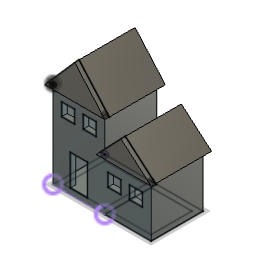
MMEZP_Domecek_3_Pokoje v1 (Autodesk Fusion 360 design; units mm, degrees)
Autodesk Fusion 360 part; units mm, degrees
sketch "Sketch1" plane through (0, 0, 0) normal (0, 1, 0) x (1, 0, 0)
  line L0 (0, 0) -> (30, 0)
  line L1 (30, 0) -> (30, -30)
  line L2 (30, -30) -> (0, -30)
  line L3 (0, -30) -> (0, 0)
  line L4 (3.2, -3.2) -> (26.8, -3.2)
  line L5 (26.8, -3.2) -> (26.8, -26.8)
  line L6 (26.8, -26.8) -> (3.2, -26.8)
  line L7 (3.2, -26.8) -> (3.2, -3.2)
  line L8 (30, 0) -> (56.8, 0)
  line L9 (56.8, 0) -> (56.8, -30)
  line L10 (56.8, -30) -> (30, -30)
  line L11 (30, -30) -> (30, 0)
  line L12 (30, -3.2) -> (53.6, -3.2)
  line L13 (53.6, -3.2) -> (53.6, -26.8)
  line L14 (53.6, -26.8) -> (30, -26.8)
  dimension "d7" = 30
  dimension "d8" = 30
  dimension "d9" = 3.2
  dimension "d10" = 3.2
  dimension "d11" = 3.2
  dimension "d12" = 3.2
  dimension "d13" = 26.8
  dimension "d14" = 30
  dimension "d15" = 3.2
  dimension "d16" = 3.2
  dimension "d17" = 3.2
  constraint horizontal L0
  constraint vertical L1
  constraint horizontal L2
  constraint vertical L3
  constraint coincident L0.start L3.end
  constraint horizontal L4
  constraint vertical L5
  constraint horizontal L6
  constraint vertical L7
  constraint horizontal L8
  constraint vertical L9
  constraint horizontal L10
  constraint vertical L11
  constraint horizontal L12
  constraint vertical L13
  constraint horizontal L14
  constraint coincident L1 L12.start
  constraint coincident L1 L14.end
  measures "d7" distance of L0.start L0.end
  measures "d8" distance of L0.start L2.end
  measures "d9" distance of L0 L4
  measures "d10" distance of L1 L5
  measures "d11" distance of L2 L6
  measures "d12" distance of L3 L7
  measures "d13" distance of L0.end L8.end
  measures "d14" distance of L8.end L9.end
  measures "d15" distance of L9 L13
  measures "d16" distance of L10 L14
  measures "d17" distance of L8 L12
extrude "Extrude1" add sketch "Sketch1" along normal blind 50 contours L0 L1 L2 L3 L11 makes body 1
extrude "Extrude2" add sketch "Sketch1" along normal blind 30 contours L1 L8 L9 L10 L11 L12 L13 L14 bodies 1
sketch "Sketch2" plane through (0, 0, 30) normal (0, 0, 1) x (1, 0, 0)
  line L0 (0, 0) -> (56.8, 0)
  line L1 (56.8, 0) -> (56.8, 30)
  line L2 (56.8, 30) -> (30, 30)
  line L3 (30, 30) -> (30, 50)
  line L4 (30, 50) -> (0, 50)
  line L5 (0, 50) -> (0, 0)
  line L6 (10, 21.2) -> (20, 21.2)
  line L7 (20, 21.2) -> (20, 3.2)
  line L8 (20, 3.2) -> (10, 3.2)
  line L9 (10, 3.2) -> (10, 21.2)
  line L10 (5, 44) -> (12.5, 44)
  line L11 (12.5, 44) -> (12.5, 36.5)
  line L12 (12.5, 36.5) -> (5, 36.5)
  line L13 (5, 36.5) -> (5, 44)
  line L14 (17.5, 44) -> (25, 44)
  line L15 (25, 44) -> (25, 36.5)
  line L16 (25, 36.5) -> (17.5, 36.5)
  line L17 (17.5, 36.5) -> (17.5, 44)
  line L18 (31.8, 22) -> (39.3, 22)
  line L19 (39.3, 22) -> (39.3, 14.5)
  line L20 (39.3, 14.5) -> (31.8, 14.5)
  line L21 (31.8, 14.5) -> (31.8, 22)
  line L22 (44.3, 22) -> (51.8, 22)
  line L23 (51.8, 22) -> (51.8, 14.5)
  line L24 (51.8, 14.5) -> (44.3, 14.5)
  line L25 (44.3, 14.5) -> (44.3, 22)
  line L26 (30, 0) -> (0, 0)
  line L27 (0, 50) -> (0, 50.5)
  line L28 (30, 50) -> (32.5, 50)
  line L29 (0, 50) -> (-2.5, 50)
  line L30 (-2.5, 50) -> (15, 70)
  line L31 (15, 70) -> (32.5, 50)
  line L32 (56.8, 30) -> (59.3, 30)
  line L33 (30, 30) -> (27.5, 30)
  line L34 (27.5, 30) -> (41.8, 45)
  line L35 (41.8, 45) -> (59.3, 30)
  dimension "d22" = 7.5
  dimension "d23" = 7.5
  dimension "d24" = 7.5
  dimension "d25" = 7.5
  dimension "d26" = 5
  dimension "d27" = 5
  dimension "d28" = 6
  dimension "d29" = 6
  dimension "d30" = 18
  dimension "d31" = 10
  dimension "d32" = 3.2
  dimension "d33" = 10
  dimension "d34" = 7.5
  dimension "d35" = 7.5
  dimension "d36" = 7.5
  dimension "d37" = 7.5
  dimension "d38" = 5
  dimension "d39" = 5
  dimension "d40" = 8
  dimension "d41" = 8
  dimension "d47" = 0.5
  dimension "d48" = 2.5
  dimension "d49" = 2.5
  dimension "d50" = 20
  dimension "d51" = 17.5
  dimension "d52" = 2.5
  dimension "d53" = 2.5
  dimension "d54" = 15
  dimension "d55" = 17.5
  constraint horizontal L6
  constraint vertical L7
  constraint horizontal L8
  constraint vertical L9
  constraint horizontal L10
  constraint vertical L11
  constraint horizontal L12
  constraint vertical L13
  constraint horizontal L14
  constraint vertical L15
  constraint horizontal L16
  constraint vertical L17
  constraint horizontal L18
  constraint vertical L19
  constraint horizontal L20
  constraint vertical L21
  constraint horizontal L22
  constraint vertical L23
  constraint horizontal L24
  constraint vertical L25
  constraint coincident L4.end L5.start
  constraint vertical L27
  constraint coincident L3.end L4.start
  constraint perpendicular L3 L28
  constraint perpendicular L5 L29
  constraint coincident L1.end L2.start
  constraint perpendicular L1 L32
  constraint coincident L2.end L3.start
  constraint perpendicular L3 L33
  measures "d22" distance of L10.start L10.end
  measures "d23" distance of L14.start L14.end
  measures "d24" distance of L14.end L15.end
  measures "d25" distance of L10.start L12.end
  measures "d26" distance of L5 L13
  measures "d27" distance of L3 L15
  measures "d28" distance of L4 L10
  measures "d29" distance of L4 L14
  measures "d30" distance of L6.start L8.end
  measures "d31" distance of L6.start L6.end
  measures "d32" distance of L8 L26
  measures "d33" distance of L5 L9
  measures "d34" distance of L22.start L22.end
  measures "d35" distance of L22.end L23.end
  measures "d36" distance of L18.start L18.end
  measures "d37" distance of L18.start L20.end
  measures "d38" distance of L1 L23
  measures "d39" distance of L19 L25
  measures "d40" distance of L2 L22
  measures "d41" distance of L2 L18
  measures "d47" distance of L4.end L27.end
  measures "d48" distance of L3.end L28.end
  measures "d49" distance of L4.end L29.end
  measures "d50" distance of L4 L30.end
  measures "d51" horizontal distance of L29.end L30.end
  measures "d52" distance of L1.end L32.end
  measures "d53" distance of L2.end L33.end
  measures "d54" distance of L2 L34.end
  measures "d55" horizontal distance of L32.end L34.end
extrude "Extrude3" add sketch "Sketch1" along normal blind 3.2 contours L4 L5 L6 L7 bodies 1
extrude "Extrude4" add sketch "Sketch1" along normal blind 3.2 contours L1 L11 L12 L13 L14 bodies 1
extrude "Extrude5" add sketch "Sketch2" along normal blind 2.5 separate body contours L4 L28 L29 L30 L31 makes body 2
extrude "Extrude6" add sketch "Sketch2" along normal blind 2.5 separate body contours L2 L3 L32 L34 L35 makes body 3
extrude "Extrude7" add sketch "Sketch2" against normal blind 32.5 contours L4 L28 L29 L30 L31 bodies 1 2
extrude "Extrude8" add sketch "Sketch2" against normal blind 32.5 contours L2 L3 L32 L34 L35 bodies 1 3
extrude "Extrude9" add sketch "Sketch2" against normal blind 32.5 contours L3 L33 L34 bodies 1
extrude "Extrude10" add sketch "Sketch2" along normal blind 2.5 contours L3 L33 L34 bodies 1
extrude "Extrude11" cut sketch "Sketch2" against normal blind 3.2 contours L6 L7 L8 L9 bodies 1
extrude "Extrude12" cut sketch "Sketch2" against normal blind 30 contours L10 L11 L12 L13 | L14 L15 L16 L17 | L18 L19 L20 L21 | L22 L23 L24 L25 bodies 1
